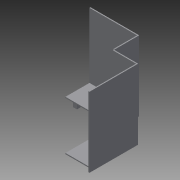
# Autodesk Inventor part: crate
Saved by Autodesk Inventor 2014 (Build 180170000, 170)
## iProperties
Created: 2015-04-09
Part Number: crate
Material: Generic
Document SubType Name: Modeling
Designer: Gus
Density: 1 g/cm^3
Appearance: Default
Author: Gus
Autodesk Inventor part; units mm, degrees
ref_plane "YZ Plane" through (0, 0, 0) normal (1, 0, 0) x (0, 1, 0)
ref_plane "XZ Plane" through (0, 0, 0) normal (0, 1, 0) x (-1, 0, 0)
ref_plane "XY Plane" through (0, 0, 0) normal (0, 0, 1) x (1, 0, 0)
sketch "Sketch1" plane through (0, 0, 0) normal (0, 1, 0) x (-1, 0, 0)
  line L0 (0, 0) -> (1206.5, 0)
  line L1 (1206.5, 0) -> (1206.5, -596.9)
  line L2 (1206.5, -596.9) -> (0, -596.9)
  line L3 (0, -596.9) -> (0, 0)
  line L4 (0, 0) -> (-596.9, 0)
  line L5 (-596.9, 0) -> (-596.9, 1206.5)
  line L6 (-596.9, 1206.5) -> (0, 1206.5)
  line L7 (0, 1206.5) -> (0, 0)
  dimension "d0" = 1206.5
  dimension "d1" = 596.9
  dimension "d2" = 596.9
  dimension "d3" = 1206.5
  constraints: 16 end point, 4 parallel, 2 horizontal, 2 perpendicular
  measures "d0" distance of L1.end L2.end
  measures "d1" distance of L0.end L1.end
  measures "d2" distance of L5.end L6.end
  measures "d3" distance of L4.end L5.end
extrude "Extrusion1" add sketch "Sketch1" along normal blind 25.4
sketch "Sketch2" plane through (0, 0, 0) normal (1, 0, 0) x (0, 1, 0)
  line L0 (0, 0) -> (1638.3, 0)
  line L1 (1638.3, 0) -> (1638.3, -618.6638)
  line L2 (1638.3, -618.6638) -> (0, -618.6638)
  line L3 (0, -618.6638) -> (0, 0)
  dimension "d6" = 1638.3
  constraints: 8 end point, 2 parallel, 1 horizontal, 1 perpendicular
  measures "d6" distance of L1.end L2.end
extrude "Extrusion2" add sketch "Sketch2" against normal blind 25.4
sketch "Sketch3" plane through (596.9, 0, 1206.5) normal (1, 0, 0) x (0, 0, -1)
  line L0 (0, 0) -> (1206.5, 0) projected
  line L1 (1206.5, 0) -> (1206.5, 25.4) projected
  line L2 (0, 25.4) -> (1206.5, 25.4) projected
  line L3 (0, 0) -> (0, 25.4) projected
  line L4 (0, 0) -> (1206.5, 0)
  line L5 (1206.5, 0) -> (1206.5, 1638.3)
  line L6 (1206.5, 1638.3) -> (0, 1638.3)
  line L7 (0, 1638.3) -> (0, 0)
  dimension "d9" = 1638.3
  constraints: 8 end point, 2 parallel, 1 horizontal, 1 perpendicular
  measures "d9" distance of L5.end L4.end
extrude "Extrusion3" add sketch "Sketch3" against normal blind 25.4 contours L7 L6 L5 L2
sketch "Sketch4" plane through (596.9, 0, 0) normal (0, 0, -1) x (-1, 0, 0)
  line L0 (0, 0) -> (596.9, 0) projected
  line L1 (596.9, 0) -> (596.9, 25.4) projected
  line L2 (25.4, 25.4) -> (596.9, 25.4) projected
  line L3 (25.4, 1638.3) -> (25.4, 25.4) projected
  line L4 (0, 1638.3) -> (25.4, 1638.3) projected
  line L5 (0, 0) -> (0, 1638.3) projected
  line L6 (0, 1638.3) -> (596.9, 1638.3)
  line L7 (596.9, 1638.3) -> (596.9, 0)
  line L8 (596.9, 0) -> (0, 0)
  line L9 (0, 0) -> (0, 1638.3)
  constraints: 8 end point, 2 parallel, 1 horizontal, 1 perpendicular
extrude "Extrusion4" add sketch "Sketch4" against normal blind 25.4 contours L2 L3 L6 L7
sketch "Sketch5" plane through (-1206.5, 0, -596.9) normal (0, 0, -1) x (-1, 0, 0)
  line L0 (-1181.1, 25.4) -> (-1181.1, 0) projected
  line L1 (-1181.1, 0) -> (0, 0) projected
  line L2 (0, 0) -> (0, 25.4) projected
  line L3 (-1181.1, 25.4) -> (0, 25.4) projected
  line L4 (-1206.5, 0) -> (0, 0)
  line L5 (0, 0) -> (0, 1638.3)
  line L6 (0, 1638.3) -> (-1206.5, 1638.3)
  line L7 (-1206.5, 1638.3) -> (-1206.5, 0)
  dimension "d14" = 1638.3
  constraints: 8 end point, 2 parallel, 1 horizontal, 1 perpendicular
  measures "d14" distance of L5.end L4.end
extrude "Extrusion5" add sketch "Sketch5" along normal blind 25.4 contours L0 L4 L7 L6 L5 L3
sketch "Sketch6" plane through (0, 0, 0) normal (0, -1, 0) x (1, 0, 0)
  line L0 (0, 0) -> (0, 1206.5) projected
  line L1 (596.9, 1206.5) -> (596.9, 0) projected
  line L2 (0, 940.6473) -> (596.9, 940.6473)
  line L3 (596.9, 940.6473) -> (596.9, 839.0473)
  line L4 (596.9, 839.0473) -> (0, 839.0473)
  line L5 (0, 839.0473) -> (0, 940.6473)
  line L6 (0, 383.1472) -> (596.9, 383.1472)
  line L7 (596.9, 383.1472) -> (596.9, 281.5472)
  line L8 (596.9, 281.5472) -> (0, 281.5472)
  line L9 (0, 281.5472) -> (0, 383.1472)
  dimension "d17" = 101.6
  dimension "d18" = 101.6
  constraints: 16 end point, 4 parallel, 4 point on line, 2 horizontal, 2 perpendicular
  measures "d17" distance of L2.end L3.end
  measures "d18" distance of L6.end L7.end
extrude "Extrusion6" add sketch "Sketch6" along normal blind 101.6 contours L0 L6 L1 L8 | L0 L2 L1 L4
sketch "Sketch7" plane through (0, 0, 0) normal (0, -1, 0) x (1, 0, 0)
  line L0 (-1206.5, -596.9) -> (-25.4, -596.9)
  line L1 (-25.4, -596.9) -> (-25.4, -622.3)
  line L2 (-25.4, -622.3) -> (-1206.5, -622.3)
  line L3 (-1206.5, -622.3) -> (-1206.5, -596.9)
  constraints: 8 end point, 2 parallel, 1 horizontal, 1 perpendicular
extrude "Extrusion7" add sketch "Sketch7" along normal blind 6.35
sketch "Sketch8" plane through (0, 0, 0) normal (0, -1, 0) x (1, 0, 0)
  line L0 (-1206.5, 0) -> (0, 0) projected
  line L1 (-1022.5135, 0) -> (-920.9135, 0)
  line L2 (-920.9135, 0) -> (-920.9135, -622.3)
  line L3 (-920.9135, -622.3) -> (-1022.5135, -622.3)
  line L4 (-1022.5135, -622.3) -> (-1022.5135, 0)
  line L5 (-361.5569, 0) -> (-259.9569, 0)
  line L6 (-259.9569, 0) -> (-259.9569, -622.3)
  line L7 (-259.9569, -622.3) -> (-361.5569, -622.3)
  line L8 (-361.5569, -622.3) -> (-361.5569, 0)
  dimension "d23" = 101.6
  dimension "d24" = 101.6
  constraints: 16 end point, 4 parallel, 2 horizontal, 2 perpendicular, 2 point on line
  measures "d23" distance of L2.end L3.end
  measures "d24" distance of L6.end L7.end
extrude "Extrusion8" add sketch "Sketch8" along normal blind 101.6
sketch "Sketch9" plane through (596.9, 1638.3, 1206.5) normal (1, 0, 0) x (0, 0, -1)
  line L0 (0, -1638.3) -> (1206.5, -1638.3)
  line L1 (1206.5, -1638.3) -> (1206.5, -1739.9)
  line L2 (1206.5, -1739.9) -> (0, -1739.9)
  line L3 (0, -1739.9) -> (0, -1638.3)
  constraints: 8 end point, 2 parallel, 1 horizontal, 1 perpendicular
extrude "Extrusion9" add sketch "Sketch9" against normal blind 25.4
sketch "Sketch10" plane through (0, 0, 0) normal (1, 0, 0) x (0, 0, -1)
  line L0 (0, 0) -> (622.3, 0)
  line L1 (622.3, 0) -> (622.3, -101.6)
  line L2 (622.3, -101.6) -> (0, -101.6)
  line L3 (0, -101.6) -> (0, 0)
  dimension "d29" = 101.6
  constraints: 8 end point, 2 parallel, 1 horizontal, 1 perpendicular
  measures "d29" distance of L0.end L1.end
extrude "Extrusion10" add sketch "Sketch10" against normal blind 25.4
sketch "Sketch11" plane through (596.9, 1638.3, 0) normal (0, 0, -1) x (-1, 0, 0)
  line L0 (0, -1739.9) -> (596.9, -1739.9)
  line L1 (596.9, -1739.9) -> (596.9, -1638.3)
  line L2 (596.9, -1638.3) -> (0, -1638.3)
  line L3 (0, -1638.3) -> (0, -1739.9)
  constraints: 8 end point, 2 parallel, 1 horizontal, 1 perpendicular
extrude "Extrusion11" add sketch "Sketch11" against normal blind 25.4
sketch "Sketch12" plane through (-1206.5, 0, -622.3) normal (0, 0, -1) x (-1, 0, 0)
  line L0 (-1181.1, 25.4) -> (0, 25.4)
  line L1 (0, 25.4) -> (0, -101.6)
  line L2 (0, -101.6) -> (-1181.1, -101.6)
  line L3 (-1181.1, -101.6) -> (-1181.1, 25.4)
  point P0 (-1206.5, 0)
  constraints: 8 end point, 2 parallel, 1 horizontal, 1 perpendicular
extrude "Extrusion12" add sketch "Sketch12" against normal blind 25.4
body "Solid1"
